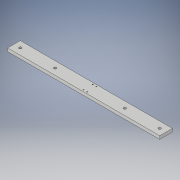
# Autodesk Inventor part: table reinforcement
Saved by Autodesk Inventor 2018 (Build 220112000, 112)
## iProperties
Created: 2018-11-15
Part Number: table reinforcement
Material: Generic
Document SubType Name: Modeling
Designer: Admin
Density: 1 g/cm^3
Appearance: Default
Author: Admin
Autodesk Inventor part; units mm, degrees
ref_plane "YZ Plane" through (0, 0, 0) normal (1, 0, 0) x (0, 1, 0)
ref_plane "XZ Plane" through (0, 0, 0) normal (0, 1, 0) x (-1, 0, 0)
ref_plane "XY Plane" through (0, 0, 0) normal (0, 0, 1) x (1, 0, 0)
sketch "Sketch1" plane through (0, 0, 0) normal (0, 1, 0) x (-1, 0, 0)
  line L0 (304.8, 25.4) -> (-304.8, 25.4)
  line L1 (-304.8, 25.4) -> (-304.8, -25.4)
  line L2 (-304.8, -25.4) -> (304.8, -25.4)
  line L3 (304.8, -25.4) -> (304.8, 25.4)
  line L4 (304.8, 25.4) -> (-304.8, -25.4) construction
  line L5 (-304.8, 25.4) -> (304.8, -25.4) construction
  point P0 (0, 0)
  dimension "d0" = 609.6
  dimension "d1" = 50.8
  constraints: 12 end point, 2 midpoint, 2 parallel, 1 horizontal, 1 perpendicular
  measures "d0" distance of L2.end L1.end
  measures "d1" distance of L1.end L0.end
extrude "Extrusion1" add sketch "Sketch1" along normal blind 12.7
sketch "Sketch2" plane through (0, 12.7, 0) normal (0, 1, 0) x (1, 0, 0)
  line L0 (0, 0) -> (0, 46.0964) construction
  line L1 (0, 0) -> (279.4, 0) construction
  line L2 (0, 0) -> (139.7, 0) construction
  point P0 (-139.7, 0)
  point P1 (-279.4, 0)
  dimension "d4" = 279.4
  dimension "d5" = 139.7
  constraints: 6 end point, 2 coincident, 2 symmetric about line, 1 horizontal, 1 midpoint, 1 vertical
  measures "d4" distance of L0.start L1.end
  measures "d5" distance of L0.start L2.end
hole "Hole1" at (139.7, 12.7, 0) at (279.4, 12.7, 0) at (-139.7, 12.7, 0) at (-279.4, 12.7, 0) direction (0, -1, 0) diameter 10.0838 end through all clearance for "Flat Head Machine Screw (82)" size "3/8" standard "Ansi Unified Screw Threads"
sketch "Sketch3" plane through (0, 12.7, 0) normal (0, 1, 0) x (1, 0, 0)
  line L0 (7.3025, 18.161) -> (-7.3025, 18.161) construction
  line L1 (-7.3025, 18.161) -> (-7.3025, -18.161) construction
  line L2 (-7.3025, -18.161) -> (7.3025, -18.161) construction
  line L3 (7.3025, -18.161) -> (7.3025, 18.161) construction
  line L4 (7.3025, 18.161) -> (-7.3025, -18.161) construction
  line L5 (-7.3025, 18.161) -> (7.3025, -18.161) construction
  point P0 (0, 0)
  dimension "d13" = 14.605
  dimension "d14" = 36.322
  constraints: 12 end point, 4 coincident, 2 midpoint, 2 parallel, 1 horizontal, 1 perpendicular
  measures "d13" distance of L2.end L1.end
  measures "d14" distance of L1.end L0.end
hole "Hole2" at (-7.3025, 12.7, -18.161) at (7.3025, 12.7, -18.161) at (7.3025, 12.7, 18.161) at (-7.3025, 12.7, 18.161) direction (0, -1, 0) diameter 3.9624 end through all thread size "10-32 UNF" class "2B" standard "ANSI Unified Screw Threads"
body "Solid1"
